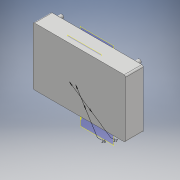
# Autodesk Inventor part: NespressoSpeedfiller-6x-base
Saved by Autodesk Inventor 2017 (Build 210142000, 142)
## iProperties
Created: 2018-08-27
Part Number: NespressoSpeedfiller-6x-base
Material: Generic
Document SubType Name: Modeling
Designer: 45027374
Density: 1 g/cm^3
Appearance: Default
Author: 45027374
Autodesk Inventor part; units mm, degrees
ref_plane "YZ Plane" through (0, 0, 0) normal (1, 0, 0) x (0, 1, 0)
ref_plane "XY Plane" through (0, 0, 0) normal (0, 0, 1) x (1, 0, 0)
sketch "Sketch1" plane through (0, 0, 0) normal (0, 1, 0) x (-1, 0, 0)
  line L0 (25.9, 0) -> (-25.9, 0) projected
  line L1 (0, -25.9) -> (0, 25.9) projected
  circle A0 centre (0, 0) radius 18.5 construction
  circle A1 centre (0, 0) radius 13 construction
  dimension "d0" = 37
  dimension "d1" = 26
  constraints: 2 centre point, 2 coincident
  measures "d0" diameter of A0
  measures "d1" diameter of A1
sketch "Sketch2" plane through (0, 0, 0) normal (0, 1, 0) x (-1, 0, 0)
  line L0 (88.2, 0) -> (-88.2, 0) projected
  line L1 (0, -36.8) -> (0, 73.8) projected
  line L2 (-63, 58) -> (-63, -21)
  line L3 (-63, -21) -> (63, -21)
  line L4 (63, -21) -> (63, 58)
  line L5 (-63, 58) -> (63, 58)
  circle A0 centre (0, 37) radius 18.5 construction
  point P0 (0, 0)
  dimension "d3" = 126
  dimension "d29" = 21
  dimension "d30" = 58
  dimension "d149" = 37
  dimension "d150" = 37
  constraints: 8 end point, 1 centre point, 1 horizontal, 1 parallel, 1 point on line, 1 other
  measures "d3" distance of L2.end L3.end
  measures "d29" distance between parallel lines of L0 L3
  measures "d30" distance between parallel lines of L5 L0
  measures "d149" diameter of A0
  measures "d150" distance of point (0, 0) A0.centre
extrude "Extrusion1" add sketch "Sketch2" along normal blind 22
sketch "Sketch8" plane through (0, 0, 0) normal (0, 1, 0) x (-1, 0, 0)
  circle A0 centre (0, 0) radius 12.25
  dimension "d34" = 24.5
  constraints: 1 centre point, 1 coincident
  measures "d34" diameter of A0
sketch "Sketch9" plane through (0, 22, 0) normal (0, 1, 0) x (1, 0, 0)
  circle A0 centre (0, 0) radius 13
  circle A1 centre (0, 0) radius 15
  dimension "d40" = 26
  dimension "d41" = 30
  constraints: 2 centre point, 2 coincident
  measures "d40" diameter of A0
  measures "d41" diameter of A1
extrude "Extrusion10" [suppressed]
sketch "Sketch10" plane through (0, 5, 0) normal (0, 1, 0) x (1, 0, 0)
  arc A0 (16, 0) -> (-16, 0) centre (0, 0) ccw projected
  line L0 (1.5, -18) -> (-1.5, -18)
  line L1 (-29.4, 0) -> (29.4, 0) projected
  line L2 (0, 36.3) -> (0, -70.8) projected
  line L3 (1.5, -12) -> (-1.5, -12)
  line L4 (1.5, -12) -> (1.5, -18)
  line L5 (-1.5, -18) -> (-1.5, -12)
  dimension "d48" = 3
  dimension "d49" = 12
  dimension "d50" = 6
  constraints: 8 end point, 2 perpendicular, 1 horizontal, 1 parallel, 1 other
  measures "d48" distance between parallel lines of L4 L5
  measures "d49" distance between parallel lines of L1 L3
  measures "d50" distance between parallel lines of L0 L3
extrude "Extrusion11" [suppressed]
ref_plane "Work Plane1" through (0, 5, 0) normal (0, 1, 0) x (-1, 0, 0)
fillet "Fillet3" radius 2 2 edges at (63, 11, 58) (-63, 11, 58)
ref_plane "Work Plane2" through (0, 22, 0) normal (0, 1, 0) x (-1, 0, 0)
sketch "Sketch16" plane through (0, 22, 0) normal (0, 1, 0) x (-1, 0, 0)
  line L0 (25.9, 0) -> (-25.9, 0) projected
  line L1 (0, -25.9) -> (0, 25.9) projected
  circle A0 centre (0, 0) radius 13.75
  dimension "d97" = 27.5
  constraints: 1 centre point, 1 coincident
  measures "d97" diameter of A0
loft "Loft1" cut profiles "Sketch8", "Sketch16"
pattern_linear "Rectangular Pattern2" count 2 spacing 37 along (0, 0, 1) count 3 spacing 37 along (1, 0, 0) of "Loft1" second direction both ways yes
sketch "Sketch17" plane through (0, 0, 0) normal (0, 1, 0) x (-1, 0, 0)
  line L0 (-63, 58) -> (63, 58)
  line L1 (63, 58) -> (63, -21)
  line L2 (63, -21) -> (-63, -21)
  line L3 (-63, -21) -> (-63, 58)
  line L4 (88.2, 0) -> (-88.2, 0) projected
  line L5 (0, -36.3) -> (0, 70.8) projected
  point P0 (0, 0)
  dimension "d105" = 21
  dimension "d106" = 58
  dimension "d107" = 126
  constraints: 8 end point, 2 parallel, 1 horizontal, 1 perpendicular, 1 other
  measures "d105" distance between parallel lines of L2 L4
  measures "d106" distance between parallel lines of L0 L4
  measures "d107" distance between parallel lines of L1 L3
extrude "Extrusion18" add sketch "Sketch17" against normal blind 2
fillet "Fillet8" radius 2 2 edges at (63, -1, 58) (-63, -1, 58)
sketch "Sketch18" plane through (0, 0, 0) normal (1, 0, 0) x (0, 1, 0)
  line L0 (22, -21) -> (0, -21)
  line L1 (0, -21) -> (0, -51)
  line L2 (0, -51) -> (22, -51)
  line L3 (22, -51) -> (22, -21)
  line L4 (20, -23) -> (2, -23)
  line L5 (2, -23) -> (2, -49)
  line L6 (2, -49) -> (20, -49)
  line L7 (20, -49) -> (20, -23)
  line L8 (-4.4, 0) -> (26.4, 0) projected
  line L9 (0, -64.9) -> (0, 32.4) projected
  point P0 (0, 0)
  dimension "d119" = 21
  dimension "d120" = 51
  dimension "d121" = 22
  dimension "d122" = 2
  dimension "d123" = 23
  dimension "d124" = 20
  dimension "d125" = 49
  constraints: 16 end point, 4 parallel, 2 horizontal, 2 perpendicular, 1 collinear
  measures "d119" distance between parallel lines of L8 L0
  measures "d120" distance between parallel lines of L8 L2
  measures "d121" distance between parallel lines of L3 L1
  measures "d122" distance between parallel lines of L9 L5
  measures "d123" distance between parallel lines of L8 L4
  measures "d124" distance between parallel lines of L1 L7
  measures "d125" distance between parallel lines of L8 L6
extrude "Extrusion20" [suppressed]
fillet "Fillet10" [suppressed]
fillet "Fillet11" radius 2 2 edges at (63, 10, -21) (-63, 10, -21)
sketch "Sketch20" plane through (0, 22, 0) normal (0, 1, 0) x (-1, 0, 0)
  circle A0 centre (-52.75, 55.5) radius 2.5
  line L0 (88.2, 0) -> (-88.2, 0) projected
  line L1 (0, -36.8) -> (0, 73.8) projected
  line L2 (73.3227, 55.5) -> (-69.7714, 55.5) construction
  line L3 (-52.75, 70.3981) -> (-52.75, -61.6245) construction
  circle A1 centre (-52.75, 18.5) radius 2.5
  circle A2 centre (-52.75, -18.5) radius 2.5
  circle A3 centre (52.75, 55.5) radius 2.5
  circle A4 centre (52.75, 18.5) radius 2.5
  circle A5 centre (52.75, -18.5) radius 2.5
  point P0 (0, 0)
  dimension "d151" = 55.5
  dimension "d152" = 52.75
  dimension "d153" = 5
  dimension "d156" = 37
  dimension "d159" = 105.5
  constraints: 6 centre point, 4 end point, 2 horizontal, 2 point on line, 2 vertical, 10 other
  measures "d151" distance between parallel lines of L0 L2
  measures "d152" distance between parallel lines of L1 L3
  measures "d153" diameter of A0
  measures "d156" distance of A0.centre A1.centre
  measures "d159" distance of A0.centre A3.centre
extrude "Extrusion22" add sketch "Sketch20" along normal blind 5
body "Solid1"
